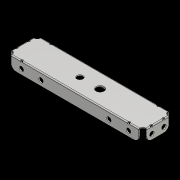
# Autodesk Inventor part: back
Saved by Autodesk Inventor 2018.2 (Build 222227000, 227)
## iProperties
Created: 2019-11-16
Part Number: back
Material: アルミニウム 6061
Document SubType Name: Sheet Metal
Designer: gisen
Density: 2.7 g/cm^3
Sheet Metal Rule: Default_mm
Appearance: アルミニウム - フラット
Author: gisen
Autodesk Inventor part; units mm, degrees
ref_plane "YZ Plane" through (0, 0, 0) normal (1, 0, 0) x (0, 1, 0)
ref_plane "XZ Plane" through (0, 0, 0) normal (0, 1, 0) x (-1, 0, 0)
ref_plane "XY Plane" through (0, 0, 0) normal (0, 0, 1) x (1, 0, 0)
sketch "スケッチ1" plane through (0, 0, 0) normal (0, 0, 1) x (1, 0, 0)
  line L0 (-67.5, -15) -> (67.5, -15)
  line L1 (67.5, -15) -> (67.5, 15)
  line L2 (67.5, 15) -> (-67.5, 15)
  line L3 (-67.5, 15) -> (-67.5, -15)
  line L4 (-67.5, -15) -> (67.5, 15) construction
  line L5 (67.5, -15) -> (-67.5, 15) construction
  line L6 (-67.5, 11) -> (-63.5, 11)
  line L7 (-63.5, 11) -> (-63.5, 15)
  line L8 (-67.5, -11) -> (-63.5, -11)
  line L9 (-63.5, -11) -> (-63.5, -15)
  line L10 (63.5, 15) -> (63.5, 11)
  line L11 (63.5, 11) -> (67.5, 11)
  line L12 (67.5, -11) -> (63.5, -11)
  line L13 (63.5, -11) -> (63.5, -15)
  point P0 (0, 0)
  dimension "d0" = 135
  dimension "d1" = 30
  dimension "d2" = 4
  measures "d0" distance of L1.end L2.end
  measures "d1" distance of L0.end L1.end
  measures "d2" distance of L6.end L7.end
extrude "プレート1" add sketch "スケッチ1" along normal blind 1 contours L9 L8 L3 L6 L7 L2 L10 L11 L1 L12 L13 L0
sketch "スケッチ2" plane through (63.5, 14, 1) normal (0, 1, 0) x (-1, 0, 0)
  line L0 (127, 0) -> (0, 0)
  line L1 (0, 0) -> (0, -12)
  line L2 (0, -12) -> (127, -12)
  line L3 (127, -12) -> (127, 0)
  constraints: 6 end point, 1 horizontal, 1 perpendicular, 1 vertical
edge flange "フランジ1" height 12 angle 90 thickness 1 bend radius 0 thickness toward (0, 1, 0) relief straight relief width 1 relief depth 0.5 corner gap 0 corner form 0 edges at (0, 15, 0) (0, -15, 0) (67.5, 0, 0) (-67.5, 0, 0) wall of the first edge with corners at (-63.5, 14, 1) (63.5, 14, 1) (63.5, 14, -11) (-63.5, 14, -11)
bend "曲げ1"
corner "コーナー1"
sketch "スケッチ3" plane through (-63.5, 15, -11) normal (0, 1, 0) x (1, 0, 0)
  line L0 (0, 0) -> (127, 0) construction
  line L1 (127, -12) -> (0, -12) construction
  line L2 (127, 0) -> (0, 0) construction
  line L3 (63.5, 0) -> (63.5, -12) construction
  line L4 (0, -12) -> (127, -12) construction
  line L5 (63.5, -5) -> (29.75, -5) construction
  line L6 (29.75, -5) -> (10.25, -5) construction
  circle A0 centre (10.25, -5) radius 2.25
  circle A1 centre (29.75, -5) radius 2.25
  circle A2 centre (116.75, -5) radius 2.25
  circle A3 centre (97.25, -5) radius 2.25
  point P0 (63.5, -11)
  dimension "d14" = 33.75
  dimension "d15" = 7
  dimension "d16" = 19.5
  dimension "d17" = 4.5
  constraints: 6 end point, 4 centre point, 2 coincident, 2 horizontal, 2 midpoint, 2 symmetric about line, 1 equal radius, 1 point on line, 2 other
  measures "d14" distance of L5.start L5.end
  measures "d15" distance between parallel lines of L1 L5
  measures "d16" distance of L5.end L6.end
  measures "d17" diameter of A0
extrude "押し出し1" cut sketch "スケッチ3" against normal through all
fillet "フィレット1" radius 5 4 edges at (-63.5, 14.5, -11) (63.5, 14.5, -11) (63.5, -14.5, -11) (-63.5, -14.5, -11)
sketch "スケッチ4" plane through (67.5, -11, -11) normal (1, 0, 0) x (0, 0, -1)
  line L0 (0, 22) -> (0, 0) construction
  line L1 (-12, 0) -> (-12, 22) construction
  line L2 (-12, 11) -> (0, 11) construction
  line L3 (-5, 22) -> (-5, 0) construction
  circle A0 centre (-5, 17) radius 2.25
  line L4 (-10.999, 22) -> (0, 22) projected
  circle A1 centre (-5, 5) radius 2.25
  point P0 (-11, 11)
  dimension "d21" = 7
  dimension "d22" = 11
  dimension "d23" = 5
  dimension "d24" = 4.5
  constraints: 4 end point, 2 centre point, 2 midpoint, 1 point on line, 1 symmetric about line, 1 vertical, 1 other
  measures "d21" distance between parallel lines of L1 L3
  measures "d22" distance between parallel lines of L2 L4
  measures "d23" distance from line of A0.centre L4
  measures "d24" diameter of A0
extrude "押し出し2" cut sketch "スケッチ4" against normal through all
fillet "フィレット2" radius 5 4 edges at (67, 11, -11) (67, -11, -11) (-67, 11, -11) (-67, -11, -11)
sketch "スケッチ5" plane through (0, 0, 1) normal (0, 0, 1) x (1, 0, 0)
  line L0 (-66.499, 11) -> (-66.499, -11) construction
  line L1 (-63.5, -11) -> (-66.499, -11) construction
  line L2 (-63.5, -13.999) -> (-63.5, -11) construction
  line L3 (-63.5, -13.999) -> (63.5, -13.999) construction
  line L4 (63.5, -11) -> (63.5, -13.999) construction
  line L5 (66.499, -11) -> (63.5, -11) construction
  line L6 (66.499, -11) -> (66.499, 11) construction
  line L7 (63.5, 11) -> (66.499, 11) construction
  line L8 (63.5, 13.999) -> (63.5, 11) construction
  line L9 (63.5, 13.999) -> (-63.5, 13.999) construction
  line L10 (-63.5, 11) -> (-63.5, 13.999) construction
  line L11 (-66.499, 11) -> (-63.5, 11) construction
  circle A0 centre (-10, 0) radius 3.055
  line L12 (-66.499, 0) -> (66.499, 0) construction
  circle A1 centre (10, 0) radius 4
  point P0 (0, 0)
  dimension "d28" = 6.11
  dimension "d29" = 10
  dimension "d30" = 8
  dimension "d31" = 10
  constraints: 2 centre point, 2 end point, 2 midpoint, 2 point on line
  measures "d28" diameter of A0
  measures "d29" distance of point (0, 0) A0.centre
  measures "d30" diameter of A1
  measures "d31" distance of A1.centre point (0, 0)
extrude "押し出し3" cut sketch "スケッチ5" against normal through all
fillet "フィレット3" radius 2.5 4 edges at (63.5, -11, 0.5) (63.5, 11, 0.5) (-63.5, 11, 0.5) (-63.5, -11, 0.5)
unfold all bends "展開1" k factor 0.44 fixed face at (3.1726, 10.6569, 1)
sketch "スケッチ6" plane through (0, 0, 1) normal (0, 0, 1) x (1, 0, 0)
  line L0 (-63.5, 14.6917) -> (63.5, 14.6917) construction
  line L1 (-63.5, 13.999) -> (-63.5, 14.6917) construction
  line L2 (63.5, 13.999) -> (-63.5, 13.999) construction
  line L3 (63.5, 14.6917) -> (63.5, 13.999) construction
  line L4 (-67.1917, -11) -> (-67.1917, 11) construction
  line L5 (-66.499, -11) -> (-67.1917, -11) construction
  line L6 (-66.499, 11) -> (-66.499, -11) construction
  line L7 (-67.1917, 11) -> (-66.499, 11) construction
  line L8 (-66.499, 0) -> (66.499, 0) construction
  line L9 (66.499, -11) -> (66.499, 11) construction
  line L10 (-63.5, 13.999) -> (63.5, 13.999) construction
  line L11 (0, 13.999) -> (0, -13.999) construction
  line L12 (-63.5, -13.999) -> (63.5, -13.999) construction
  line L13 (-67.1917, 11) -> (-66.499, 11) construction
  line L14 (-66.8454, 11) -> (-66.8454, -11) construction
  line L15 (-63.5, 14.6917) -> (-63.5, 13.999) construction
  line L16 (-63.5, 14.3454) -> (63.5, 14.3454) construction
  line L17 (63.5, 14.6917) -> (63.5, 13.999) construction
  circle A0 centre (-73.1907, 6) radius 2.25 construction
  line L18 (-73.1907, 6) -> (-66.8454, 6) construction
  circle A1 centre (-53.25, 20.6907) radius 2.25 construction
  line L19 (-53.25, 20.6907) -> (-53.25, 14.3454) construction
  circle A2 centre (-53.25, 14.3454) radius 1.1
  circle A3 centre (-66.8454, 6) radius 1.1
  circle A4 centre (-53.25, -14.3454) radius 1.1
  circle A5 centre (-66.8454, -6) radius 1.1
  circle A6 centre (53.25, 14.3454) radius 1.1
  circle A7 centre (66.8454, 6) radius 1.1
  circle A8 centre (66.8454, -6) radius 1.1
  circle A9 centre (53.25, -14.3454) radius 1.1
  point P0 (0, 0)
  dimension "d35" = 2.2
  constraints: 12 end point, 8 centre point, 8 midpoint, 6 symmetric about line, 2 coincident, 2 point on line, 1 equal radius, 1 parallel, 1 perpendicular, 6 other
  measures "d35" diameter of A2
extrude "押し出し4" cut sketch "スケッチ6" against normal up to surface (1 mm away)
refold all bends "再折り曲げ1"
equation "\"d3\" = Thickness"
equation "\"d4\" = BendReliefWidth"
equation "\"d5\" = BendReliefDepth"
equation "\"d6\" = MinimumRemnant"
equation "\"d11\" = CornerReliefSize"
equation "\"d12\" = GapSize"
equation "\"d31\" = d29"
equation "\"BendReliefWidth\" = Thickness"
equation "\"BendReliefDepth\" = 0.5 * Thickness"
equation "\"CornerReliefSize\" = 4 * Thickness"
equation "\"MinimumRemnant\" = 2 * Thickness"
equation "\"GapSize\" = Thickness"
equation "\"Thickness\" = 1"
